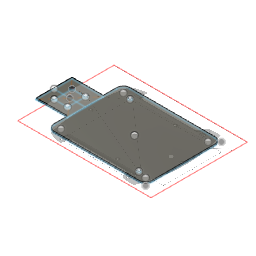
Support Throttle v3 (Autodesk Fusion 360 design; units mm, degrees)
Autodesk Fusion 360 part; units mm, degrees
sketch "Esquisse1" plane through (0, 0, 0) normal (0, 0, 1) x (1, 0, 0)
  circle A0 centre (-65, 59.5) radius 3.2016
  circle A1 centre (85, -71) radius 3.1623
  line L0 (-85, 79.25) -> (105, 79.25)
  line L1 (120, 64.25) -> (120, -75.75)
  line L2 (105, -90.75) -> (-85, -90.75)
  line L3 (-100, -75.75) -> (-100, 64.25)
  line L4 (-100, -5.75) -> (-170, -5.75)
  line L5 (-170, 34.25) -> (-100, 34.25)
  line L6 (-100, 34.25) -> (-100, -45.75)
  line L7 (-100, -45.75) -> (-170, -45.75)
  line L8 (-170, -45.75) -> (-170, 34.25)
  line L9 (-170, 34.25) -> (-100, -45.75) construction
  line L10 (-100, 34.25) -> (-170, -45.75) construction
  arc A2 (-85, 79.25) -> (-100, 64.25) centre (-85, 64.25) ccw
  arc A3 (120, 64.25) -> (105, 79.25) centre (105, 64.25) ccw
  arc A4 (105, -90.75) -> (120, -75.75) centre (105, -75.75) ccw
  arc A5 (-100, -75.75) -> (-85, -90.75) centre (-85, -75.75) ccw
  line L11 (-150, -25.75) -> (-150, 14.25)
  line L12 (-150, 14.25) -> (-120, 14.25)
  line L13 (-120, 14.25) -> (-120, -25.75)
  line L14 (-120, -25.75) -> (-150, -25.75)
  circle A6 centre (-150, 14.25) radius 4
  circle A7 centre (-120, 14.25) radius 4
  circle A8 centre (-150, -25.75) radius 4
  circle A9 centre (-120, -25.75) radius 4
  point P0 (120, 79.25)
  point P1 (120, -90.75)
  point P2 (10, -5.75)
  point P3 (-135, -5.75)
  dimension "d1" = 170
  dimension "d2" = 70
  dimension "d3" = 70
  dimension "d4" = 80
  dimension "d11" = 15
  dimension "d14" = 20
  dimension "d15" = 8
  dimension "d18" = 30
  dimension "d19" = -40
  constraint horizontal L0
  constraint perpendicular L0 L1
  constraint parallel L0 L2
  constraint parallel L1 L3
  constraint perpendicular L3 L4
  constraint horizontal L5
  constraint perpendicular L5 L6
  constraint parallel L5 L7
  constraint parallel L6 L8
  constraint coincident L9 P3
  constraint coincident L10 P3
  constraint midpoint L4 P3
  constraint coincident L3 L4.start
  constraint tangent L0 A2
  constraint tangent L3 A2
  constraint coincident P0 L0
  constraint coincident P0 L1
  constraint tangent L0 A3
  constraint tangent L1 A3
  constraint equal A2 A3
  constraint coincident P1 L1
  constraint coincident P1 L2
  constraint tangent L1 A4
  constraint tangent L2 A4
  constraint equal A2 A4
  constraint tangent L2 A5
  constraint tangent L3 A5
  constraint equal A2 A5
  constraint coincident L11.end L12.start
  measures "d1" distance of P0 P1
  measures "d2" distance of L4.start L4.end
  measures "d3" distance of L6.end L7.end
  measures "d4" distance of L5.end L6.end
  measures "d11" radius of A2
  measures "d15" diameter of A6
extrude "Extrusion1" add sketch "Esquisse1" along normal blind 3
extrude "Extrusion2" cut sketch "Esquisse1" along normal blind 3 contours L12 L13 A7 | L12 L13 A7 | L13 L14 A9 | L13 L14 A9 | L11 L14 A8 | L11 L14 A8 | L11 L12 A6 | L11 L12 A6
